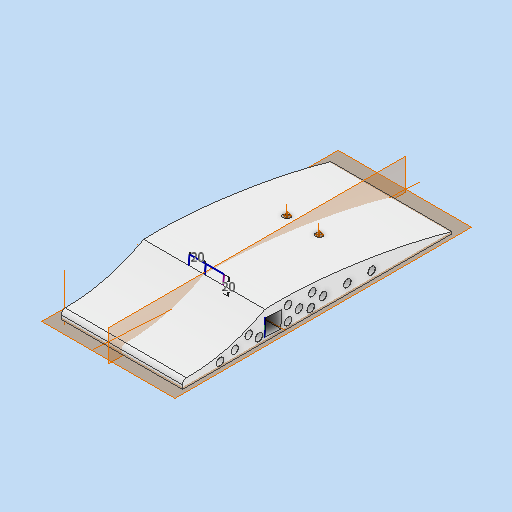
# Autodesk Inventor part: WingBox
Saved by Autodesk Inventor 2027 (Build 310192060, 192F)
## iProperties
Created: 2025-08-01
Part Number: WingBox
Material: Plastic, Opaque White
Document SubType Name: Modeling
Designer: Cupri
Density: 0.306341 g/cm^3
Appearance: Smooth - White
Mass: 301.16 g
Surface Area: 1355.43 cm^2
Volume: 983.088 cm^3
Author: Cupri
## iProperties of the stored document WingBox_3DPrint.ipt
Created: 2025-08-03
Part Number: WingBox_3DPrint
Material: Generic
Document SubType Name: Modeling
Designer: Cupri
Density: 1 g/cm^3
Appearance: Default
Author: Cupri
Autodesk Inventor part; units mm, degrees
ref_plane "YZ Plane" through (0, 0, 0) normal (1, 0, 0) x (0, 1, 0)
ref_plane "XY Plane" through (0, 0, 0) normal (0, 0, 1) x (1, 0, 0)
sketch "Sketch1" plane through (0, 0, 0) normal (1, 0, 0) x (0, 1, 0)
  line L0 (-2.1632, -329.9963) -> (-0.9745, -330.0014)
  line L1 (-2.1632, -329.9951) -> (-2.1632, -329.9963)
  line L2 (-2.1632, -329.9951) -> (-2.4422, -329.9951)
  spline S0 degree 3 poles (-0.405, -330.1552) (0.9537, -325.1233) (1.9563, -321.5105) (2.8807, -318.1296) (3.8079, -314.7389) (4.6565, -311.5815) (5.583, -307.9714) (6.5095, -304.3611) (7.5137, -300.2982) (8.6298, -295.6026) (9.7548, -290.8694) (10.9937, -285.4924) (12.2548, -279.8086) (13.5479, -273.9809) (14.8422, -267.9178) (16.0284, -262.0542) (17.2338, -256.0958) (18.3276, -250.3438) (19.3395, -244.7228) (20.6698, -237.333) (21.892, -230.0631) (23.0732, -222.6141) (24.654, -212.6457) (26.1278, -202.3745) (27.3659, -192.1289) (28.2425, -184.8742) (29.0102, -177.6615) (29.6986, -170.63) (30.3698, -163.7739) (30.9693, -157.1031) (31.4539, -150.2338) (31.8154, -145.1091) (32.1063, -139.8058) (32.3036, -134.2671) (32.5007, -128.7338) (32.6046, -122.9656) (32.6262, -117.43) (32.6455, -112.4952) (32.603, -107.8232) (32.5118, -103.6944) (32.4197, -99.5266) (32.278, -95.9127) (32.0844, -92.603) (31.8816, -89.1345) (31.6185, -85.9081) (31.2933, -82.5398) (30.931, -78.7879) (30.4919, -74.8552) (30.0019, -70.9506) (29.515, -67.0719) (28.9863, -63.3007) (28.3579, -59.5488) (27.8334, -56.4177) (27.2229, -53.2286) (26.4972, -49.8793) (25.6301, -45.8774) (24.5968, -41.6418) (23.6015, -37.941) (22.8353, -35.0925) (22.1029, -32.6059) (21.4229, -30.4603) (20.5882, -27.827) (19.838, -25.6271) (18.984, -23.281) (18.321, -21.4595) (17.5736, -19.5423) (16.6309, -17.484) (15.7038, -15.4598) (14.5791, -13.2961) (13.5588, -11.4077) (12.7581, -9.9257) (12.0684, -8.6632) (11.4412, -7.6048) (10.7635, -6.4611) (10.1286, -5.5191) (9.1146, -4.4162) (8.2619, -3.4886) (7.1303, -2.4284) (5.764, -1.4444) (4.4879, -0.5254) (3.0248, 0.2881) (1.5908, 0.5476) (0.3755, 0.7675) (-0.8188, 0.5632) (-1.8076, 0.0108) (-3.0331, -0.6739) (-3.9409, -1.785) (-4.6412, -2.8204) (-5.3573, -3.879) (-5.8545, -4.8644) (-6.2513, -5.8012) (-6.7038, -6.8694) (-7.0446, -7.9661) (-7.4083, -9.3616) (-7.9306, -11.3656) (-8.5009, -13.9974) (-8.9016, -16.5042) (-9.2532, -18.7033) (-9.4614, -20.7666) (-9.6076, -22.6841) (-9.8004, -25.2116) (-9.9342, -27.5205) (-10.0673, -30.276) (-10.1703, -32.4093) (-10.2532, -34.8679) (-10.2982, -37.6909) (-10.3544, -41.2137) (-10.3539, -45.2486) (-10.3194, -49.0894) (-10.289, -52.4587) (-10.2331, -55.6701) (-10.1531, -58.7874) (-10.0605, -62.4007) (-9.9312, -65.9923) (-9.7768, -69.6992) (-9.6107, -73.6891) (-9.4198, -77.7513) (-9.2427, -81.6143) (-9.0879, -84.9923) (-8.9437, -88.2148) (-8.7967, -91.6207) (-8.6574, -94.8459) (-8.5102, -98.3178) (-8.3389, -102.3319) (-8.1674, -106.351) (-7.9717, -110.9139) (-7.7658, -115.7923) (-7.5352, -121.2588) (-7.2978, -127.0252) (-7.0821, -132.579) (-6.8662, -138.1406) (-6.672, -143.4886) (-6.4924, -148.6356) (-6.2558, -155.4121) (-6.0346, -161.9593) (-5.7967, -168.6776) (-5.4813, -177.5831) (-5.1373, -186.7926) (-4.8158, -196.0325) (-4.5204, -204.5215) (-4.2474, -213.0024) (-4.0058, -221.2906) (-3.7869, -228.8022) (-3.5917, -236.1329) (-3.4197, -243.5699) (-3.2893, -249.2072) (-3.1723, -254.9654) (-3.0688, -260.9509) (-2.9665, -266.8676) (-2.8774, -273.0072) (-2.8015, -278.9371) (-2.7285, -284.6426) (-2.6679, -290.0685) (-2.6193, -294.8554) (-2.5708, -299.6265) (-2.5341, -303.7632) (-2.5074, -307.4316) (-2.4807, -311.1183) (-2.464, -314.3315) (-2.4544, -317.7705) (-2.4448, -321.2094) (-2.4422, -324.8742) (-2.4422, -329.9951) knots 0 0 0 0 0.019596 0.019596 0.019596 0.03925 0.03925 0.03925 0.058905 0.058905 0.058905 0.078717 0.078717 0.078717 0.099031 0.099031 0.099031 0.119673 0.119673 0.119673 0.146811 0.146811 0.146811 0.183127 0.183127 0.183127 0.208842 0.208842 0.208842 0.233915 0.233915 0.233915 0.25262 0.25262 0.25262 0.271307 0.271307 0.271307 0.287966 0.287966 0.287966 0.304782 0.304782 0.304782 0.322404 0.322404 0.322404 0.342033 0.342033 0.342033 0.361532 0.361532 0.361532 0.377805 0.377805 0.377805 0.397248 0.397248 0.397248 0.412214 0.412214 0.412214 0.430582 0.430582 0.430582 0.444843 0.444843 0.444843 0.458868 0.458868 0.458868 0.469875 0.469875 0.469875 0.48177 0.48177 0.48177 0.491774 0.491774 0.491774 0.501117 0.501117 0.501117 0.509034 0.509034 0.509034 0.518847 0.518847 0.518847 0.52888 0.52888 0.52888 0.540322 0.540322 0.540322 0.556753 0.556753 0.556753 0.571169 0.571169 0.571169 0.590171 0.590171 0.590171 0.604883 0.604883 0.604883 0.623242 0.623242 0.623242 0.639347 0.639347 0.639347 0.658015 0.658015 0.658015 0.678109 0.678109 0.678109 0.695679 0.695679 0.695679 0.712317 0.712317 0.712317 0.728976 0.728976 0.728976 0.747644 0.747644 0.747644 0.766338 0.766338 0.766338 0.79095 0.79095 0.79095 0.823575 0.823575 0.823575 0.853549 0.853549 0.853549 0.880715 0.880715 0.880715 0.901306 0.901306 0.901306 0.921661 0.921661 0.921661 0.941246 0.941246 0.941246 0.960766 0.960766 0.960766 0.980383 0.980383 0.980383 1 1 1 1
  line L3 (-0.9745, -330.0014) -> (-0.405, -330.1552)
  line L4 (2.7426, -96.8641) -> (1.6145, -117.0737)
  line L5 (1.6145, -117.0737) -> (21.8499, -118.2211)
  line L6 (21.8499, -118.2211) -> (22.9968, -97.9947)
  line L7 (22.9968, -97.9947) -> (2.7426, -96.8641)
  line L8 (-2.4422, -329.9951) -> (-2.4422, -0.3997)
  line L9 (-2.4422, -0.3997) -> (-2.4422, 4.6003)
  line L10 (-2.4422, 4.6003) -> (2.4819, 4.6003)
  arc A0 (7.4818, -0.4128) -> (32.3222, -97.4722) centre (207.4812, -0.9354) ccw
  arc A1 (7.4818, -0.4128) -> (2.4819, 4.6003) centre (2.4819, -0.3997) ccw
  line L11 (22.9968, -97.9947) -> (2.8257, -96.9376)
  line L12 (22.4233, -108.1079) -> (2.1786, -106.9689) construction
  line L13 (11.7322, -117.6474) -> (12.8697, -97.4294) construction
  point P0 (7.5578, 4.6003)
  dimension "d12" = 5
  dimension "d13" = 10
  dimension "d14" = 200
  dimension "d15" = 5
  constraints: 28 end point, 5 point on circle, 4 midpoint, 2 centre point, 2 tangent, 2 vertical, 1 horizontal, 1 point on line, 4 other
  measures "d12" distance of L8.end L9.end
  measures "d13" distance of L9.end point (7.558, 4.6)
  measures "d14" radius of A0
  measures "d15" radius of A1
extrude "Extrusion1" add sketch "Sketch1" along normal blind 150 contours L2 L8 S0 A0 L3 L0 | L9 L10 A1 A0 S0
sketch "Sketch4" plane through (0, -2.4422, -329.9951) normal (0, -1, 0) x (1, 0, 0)
  line L0 (0, 232.0004) -> (150, 232.0004) construction
  line L1 (0, 232.0004) -> (0, 211.774) construction
  line L2 (0, 211.774) -> (150, 211.774) construction
  line L3 (150, 232.0004) -> (150, 211.774) construction
  line L4 (105.25, 231.8872) -> (44.75, 231.8872)
  line L5 (44.75, 231.8872) -> (44.75, 161.3872)
  line L6 (44.75, 161.3872) -> (105.25, 161.3872)
  line L7 (105.25, 161.3872) -> (105.25, 231.8872)
  point P0 (0, 329.9951)
  point P1 (75, 99.6949)
  point P2 (150, 221.8872)
  dimension "d37" = 60.5
  dimension "d38" = 70.5
  dimension "d40" = 30.25
  dimension "d41" = 10
  constraints: 8 end point, 2 parallel, 1 horizontal, 1 midpoint, 1 perpendicular
  measures "d37" distance of L6.end L5.end
  measures "d38" distance of L5.end L4.end
  measures "d40" distance from line of point (75, 99.695) L5
  measures "d41" distance from line of point (150, 221.887) L4
extrude "Extrusion4" cut sketch "Sketch4" against normal blind 5
sketch "Sketch5" plane through (0, -2.4422, -329.9951) normal (0, -1, 0) x (1, 0, 0)
  line L0 (64.875, 161.9157) -> (85.125, 161.9157) projected
  line L1 (85.125, 161.9157) -> (85.125, 6.5707) projected
  line L2 (64.875, 6.5707) -> (85.125, 6.5707) projected
  line L3 (64.875, 6.5707) -> (64.875, 161.9157) projected
  line L4 (85.125, 100.2234) -> (64.875, 100.2234) projected
  line L5 (105.25, 212.8679) -> (105.25, 161.3872) projected
  line L6 (105.25, 161.3872) -> (44.75, 161.3872)
  line L7 (44.75, 161.3872) -> (44.75, 99.6949)
  line L8 (44.75, 99.6949) -> (105.25, 99.6949)
  line L9 (105.25, 99.6949) -> (105.25, 161.3872)
  point P0 (0, 329.9951)
  point P1 (64.875, 100.2234)
  point P2 (85.125, 100.2234)
  point P3 (64.875, 99.6949)
  point P4 (64.875, 161.3872)
  point P5 (85.125, 99.6949)
  point P6 (85.125, 161.3872)
  constraints: 8 end point, 2 parallel, 1 horizontal, 1 perpendicular
extrude "Extrusion5" cut sketch "Sketch5" against normal blind 5 contours L6 L1 L4 L3 | L3 L8 L7 L6 | L6 L9 L8 L1
sketch "Sketch6" plane through (0, 2.5578, -329.9951) normal (0, -1, 0) x (1, 0, 0)
  circle A0 centre (95, 110.7234) radius 2.75
  line L0 (85.125, 100.2234) -> (64.875, 100.2234) projected
  line L1 (75, 100.2234) -> (75, 231.8872) construction
  line L2 (44.75, 231.8872) -> (105.25, 231.8872) projected
  circle A1 centre (55, 110.7234) radius 2.75
  point P0 (0, 329.9951)
  point P1 (105.25, 100.2234)
  point P2 (44.75, 100.2234)
  dimension "d46" = 5.5
  dimension "d48" = 20
  dimension "d49" = 10.5
  constraints: 2 centre point, 2 end point, 2 midpoint, 1 symmetric about line, 1 other
  measures "d46" diameter of A0
  measures "d48" distance from line of L1 A0.centre
  measures "d49" distance from line of L0 A0.centre
hole "Hole1" at (55, 23.5974, -219.2718) direction (0, -1, 0) diameter 5.5 end through all start extended yes counterbore diameter 8.5 counterbore depth 15
hole "Hole2" at (95, 23.5974, -219.2718) direction (0, -1, 0) diameter 5.5 end through all start extended yes counterbore diameter 8.5 counterbore depth 15
ref_plane "Work Plane1" through (75, 0, 0) normal (1, 0, 0) x (0, 0, -1)
sketch "Sketch7" plane through (0, 0, 0) normal (-1, 0, 0) x (0, 0, 1)
  line L0 (-117.6238, 2.5578) -> (-117.7088, 22.3958) projected
  line L1 (-96.8641, 2.7426) -> (-97.9947, 22.9968) projected
  line L2 (-117.7088, 22.3958) -> (-96.8641, 2.7426) construction
  point P0 (0, 0)
  point P1 (-107.3342, 12.6142)
  constraints: 2 end point, 1 point on line
sketch "Sketch8" plane through (150, 2.7426, -96.8641) normal (0, -0.0557338, -0.9984457) x (-1, 0, 0)
  line L0 (150, 9.8595) -> (150, 29.5675) projected
  line L1 (150, 29.5675) -> (0, 29.5675) projected
  line L2 (0, 9.8595) -> (0, 29.5675) projected
  line L3 (150, 9.8595) -> (0, 9.8595) projected
  line L4 (64.875, 20.1693) -> (85.125, 0) construction
  point P0 (150, -8.137)
  point P1 (75, 10.0847)
  constraints: 2 end point, 1 midpoint, 2 other
sketch "Sketch9" plane through (150, 0, 0) normal (1, 0, 0) x (0, 0, -1)
  line L0 (329.9951, -2.4422) -> (335.7928, -2.4422)
  line L1 (335.7928, -2.4422) -> (335.7928, 0.7272)
  line L2 (335.7928, 0.7272) -> (329.9951, 0.7272)
  line L3 (329.9951, 0.7272) -> (329.9951, -2.4422)
  point P0 (0, 0)
  constraints: 8 end point, 2 parallel, 1 horizontal, 1 perpendicular
extrude "Extrusion6" cut sketch "Sketch9" against normal through all
sketch "Sketch10" plane through (150, 0, 0) normal (1, 0, 0) x (0, 0, -1)
  line L0 (-4.6003, -2.4422) -> (329.9951, -2.4422) projected
  circle A0 centre (126.2025, 22.6647) radius 4.5
  circle A1 centre (169.6663, 10.5004) radius 4.5
  circle A2 centre (154.2681, 5.1092) radius 4.5
  circle A3 centre (199.6316, 9.0586) radius 4.5
  circle A4 centre (156.1678, 21.223) radius 4.5
  circle A5 centre (229.5969, 7.6168) radius 4.5
  circle A6 centre (229.5969, 7.6168) radius 4.5
  circle A7 centre (77.5261, 14.9311) radius 4.5
  circle A8 centre (60.2702, 7.4237) radius 4.5
  circle A9 centre (90.2355, 5.982) radius 4.5
  circle A10 centre (42.1567, 3.8842) radius 4.5
  circle A11 centre (139.7009, 11.9421) radius 4.5
  circle A12 centre (126.2781, 4.9893) radius 4.5
  circle A13 centre (42.1567, 3.8842) radius 4.625
  circle A14 centre (60.2702, 7.4237) radius 4.625
  circle A15 centre (77.5261, 14.9311) radius 4.625
  circle A16 centre (90.2355, 5.982) radius 4.625
  circle A17 centre (126.2781, 4.9893) radius 4.625
  circle A18 centre (126.2025, 22.6647) radius 4.625
  circle A19 centre (139.7009, 11.9421) radius 4.625
  circle A20 centre (156.1678, 21.223) radius 4.625
  circle A21 centre (154.2681, 5.1092) radius 4.625
  circle A22 centre (169.6663, 10.5004) radius 4.625
  circle A23 centre (199.6316, 9.0586) radius 4.625
  circle A24 centre (229.5969, 7.6168) radius 4.625
  point P0 (0, 0)
  dimension "d116" = 9.25
  dimension "d117" = 9.25
  dimension "d118" = 9.25
  dimension "d119" = 9.25
  dimension "d120" = 9.25
  dimension "d121" = 9.25
  dimension "d122" = 9.25
  dimension "d123" = 9.25
  dimension "d124" = 9.25
  dimension "d125" = 9.25
  dimension "d127" = 9.25
  dimension "d129" = 9.25
  constraints: 25 centre point, 12 coincident, 26 other
  measures "d116" diameter of A13
  measures "d117" diameter of A14
  measures "d118" diameter of A15
  measures "d119" diameter of A16
  measures "d120" diameter of A17
  measures "d121" diameter of A18
  measures "d122" diameter of A19
  measures "d123" diameter of A20
  measures "d124" diameter of A21
  measures "d125" diameter of A22
  measures "d127" diameter of A23
  measures "d129" diameter of A24
extrude "Extrusion7" cut sketch "Sketch10" against normal blind 5 contours A0 | A1 | A2 | A3 | A4 | A5 | A7 | A8 | A9 | A10 | A11 | A12 | A13 | A14 | A15 | A16 | A17 | A18 | A19 | A20 | A21 | A22 | A23 | A24
mirror "Mirror1" about plane through (75, 0, 0) normal (1, 0, 0) of "Extrusion7"
fillet "Fillet1" radius 4.62 12 edges at (145, 14.9311, -72.9011) (145, 4.9893, -121.6531) (145, 7.6168, -224.9719) (145, 10.5004, -165.0413) (145, 22.6647, -121.5775) (145, 7.4237, -55.6452) (145, 5.982, -85.6105) (145, 21.223, -151.5428) (145, 9.0586, -195.0066) (145, 5.1092, -149.6431) (145, 11.9421, -135.0759) (145, 3.8842, -37.5317)
sketch "Sketch11" plane through (0, 0, 0) normal (0, 1, 0) x (-1, 0, 0)
  line L0 (-150, -329.9951) -> (0, -329.9951) projected
  line L1 (-150, 4.6003) -> (-150, -329.9951) projected
  line L2 (0, -329.9951) -> (-150, -329.9951)
  line L3 (-150, -329.9951) -> (-150, -328.9951)
  line L4 (-150, -328.9951) -> (0, -328.9951)
  line L5 (0, -328.9951) -> (0, -329.9951)
  point P0 (0, 0)
  dimension "d104" = 1
  constraints: 8 end point, 2 parallel, 1 horizontal, 1 perpendicular, 1 point on line
  measures "d104" distance of L2.end L3.end
extrude "Extrusion8" cut sketch "Sketch11" along normal mid plane 10
fillet "Fillet2" radius 4.6 12 edges at (5, 14.9311, -72.9011) (5, 4.9893, -121.6531) (5, 7.6168, -224.9719) (5, 10.5004, -165.0413) (5, 22.6647, -121.5775) (5, 7.4237, -55.6452) (5, 5.982, -85.6105) (5, 21.223, -151.5428) (5, 9.0586, -195.0066) (5, 5.1092, -149.6431) (5, 11.9421, -135.0759) (5, 3.8842, -37.5317)
sketch "Sketch12" plane through (0, 2.5578, -329.9951) normal (0, -1, 0) x (1, 0, 0)
  line L0 (0, 212.9214) -> (44.75, 212.9214) projected
  line L1 (44.75, 212.9214) -> (44.75, 162.9214)
  line L2 (44.75, 99.6949) -> (44.75, 231.8872) projected
  line L3 (44.75, 162.9214) -> (54.75, 162.9214)
  line L4 (54.75, 162.9214) -> (54.75, 212.9214)
  line L5 (54.75, 212.9214) -> (44.75, 212.9214)
  line L6 (44.75, 212.8679) -> (105.25, 212.8679) projected
  line L7 (105.25, 212.8679) -> (95.25, 212.8679)
  line L8 (95.25, 212.8679) -> (95.25, 162.8679)
  line L9 (95.25, 162.8679) -> (105.25, 162.8679)
  line L10 (105.25, 162.8679) -> (105.25, 212.8679)
  point P0 (0, 329.9951)
  point P1 (44.75, 100.2234)
  point P2 (85.125, 212.3713)
  dimension "d108" = 50
  dimension "d109" = 10
  dimension "d110" = 10
  dimension "d111" = 50
  constraints: 16 end point, 4 perpendicular, 2 parallel, 1 horizontal, 1 point on line, 1 other
  measures "d108" distance of L0.end L1.end
  measures "d109" distance of L1.end L3.end
  measures "d110" distance of L9.end L8.end
  measures "d111" distance of L8.end L7.end
extrude "Extrusion9" cut sketch "Sketch12" against normal up to surface surface through (0, 22.9968, -97.9947) normal (0, -0.9983963, 0.0566121)
sketch "Sketch13" plane through (150, 22.9968, -97.9947) normal (0, -0.0557338, -0.9984457) x (-1, 0, 0)
  line L0 (150, -20.2857) -> (150, 0) projected
  line L1 (0, -20.2857) -> (0, 0) projected
  line L2 (0, 0) -> (150, 0)
  line L3 (150, 0) -> (150, -20.2857)
  line L4 (150, -20.2857) -> (0, -20.2857)
  line L5 (0, -20.2857) -> (0, 0)
  line L6 (75, 0) -> (52.5304, 0)
  line L7 (52.5304, 0) -> (52.5304, 20)
  line L8 (52.5304, 20) -> (75, 20)
  line L9 (75, 20) -> (75, 0)
  line L10 (75, 0) -> (95, 0)
  line L11 (95, 0) -> (95, 20)
  line L12 (95, 20) -> (75, 20)
  line L13 (75, 20) -> (75, 0)
  point P0 (150, -28.4227)
  dimension "d114" = 20
  dimension "d115" = 20
  constraints: 24 end point, 6 parallel, 3 horizontal, 3 perpendicular, 1 midpoint, 1 point on line
  measures "d114" distance of L6.end L7.end
  measures "d115" distance of L12.end L11.end
body "Solid1"
